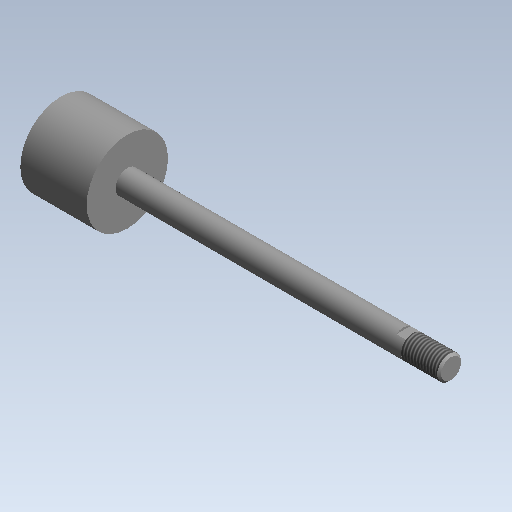
# Autodesk Inventor part: SR-092-DPY0000_rod
Saved by Autodesk Inventor 2020 (Build 240168000, 168)
## iProperties
Part Number: SR-092-DPY0000_rod
Material: Generic
Catalog Web Link: www.cadenas.de
Description: Standard Air Cylinder_rod-Original Line - Standard Air Cylinders
Vendor: BIMBA
Document SubType Name: Modeling
Designer: partserver
Manufacturer: BIMBA
Mass: 18.0803 g
Surface Area: 57.2606 cm^2
Volume: 18.0803 cm^3
Density: 1 g/cm^3
Appearance: PSOLRGB-181-181-181
Category: PARTsolutions
Company: BIMBA
PSOL_IDENT_0: {$CADENAS_DATA\23d-libs\bimba\bimba_brand\bimba_imperial\bimba_full_line\original_line_cylinders\sta
PSOL_IDENT_1: ndard_air_cylinders\rod.prj},337 {VTYP=3D},{NB=SR-092-DPY0000_rod},{LINA=SR-092-DPY0000_rod},{NN=Sta
PSOL_IDENT_2: ndard Air Cylinder_rod},{DATE=19.01.2022 10:19:37},{GEOMDATE=27.08.2019 11:00:52},{VERSION=},{LINEID=
PSOL_IDENT_3: 10},{WBVAR=STROKE,ACTING,MNT,DER,NR,BM,CO,M,EE,EEL,K,Q,Y,F,G,T,B,H,SER,SR,NT,W,E,HL,ST,STP,PRC,PB,CO
PSOL_IDENT_4: LOR1,FCD,RCD,BCD,ZHJ},{WBNUMERIC=STROKE,EEL,COLOR1,FCD,RCD,BCD,ZHJ}  {NB=SR-092-DPY0000_rod},{LINA=S
PSOL_IDENT_5: R-092-DPY0000_rod},{KT=DUMMY},{PN=SR-092-DPY000},{DASH=-},{BORE=1.06250000},{BOREPN=09},{STROKE=2.00
PSOL_IDENT_6: 0},{STROKEALG=[0.001:50/0.001]},{STROKE1=2.000},{ACTING=D},{ACTINGALG= '' , 'Single Acting' , 'R' , '
PSOL_IDENT_7: Reverse Single Acting' , 'D' , 'Double Acting' },{ACTINGPN=D},{MNT=P},{MNTALG= '' , 'Front Nose Moun
PSOL_IDENT_8: ting' , 'P' , 'Rear Pivot Mounting' , 'X' , 'Universal Pivot Mounting or Double End Mounting' , 'BF'
PSOL_IDENT_9: , 'Front Block Mounting' , 'BR' , 'Rear Block Mounting for Vertical Positioning' , 'BFT' , 'Front B
PSOL_IDENT_10: lock Trunnion Mounting' , 'BRT' , 'Rear Block Trunnion Mounting' },{TYPE=SR-},{MNTPN=P},{DER=},{DERA
PSOL_IDENT_11: LG= '' , 'N/A' },{NR=},{NRALG= '' , 'N/A' },{NRPN=},{BM=},{BMALG= '' , 'N/A' },{BMPN=},{CO=},{COALG=
PSOL_IDENT_12: '' , 'N/A' },{M=},{MALG= '', 'Without Magnet', 'M', 'With Magnet' },{EE=},{EEL=0},{EEMAX=48},{EEALG=
PSOL_IDENT_13: '', 'Without Extra Extension', 'EE', 'With Extra Extension' },{EELALG=0},{EEPN=},{EEPN1=0.000},{K=}
PSOL_IDENT_14: ,{KALG= '', 'Standard' , 'K' , 'Ports Rotated 90deg' },{KPN=},{Q=},{QALG= '' , 'Without Side Ported
PSOL_IDENT_15: Rear Head' , 'Q' , 'With Side Ported Rear Head' },{QPN=},{Y=Y},{YALG= '' , 'Without Pivot Bushing' ,
PSOL_IDENT_16: 'Y' , 'With Pivot Bushing' },{YPN=Y},{F=},{FALG= '', 'Standard', 'F', 'Molycoated Body' },{FPN=},{G=
PSOL_IDENT_17: },{GPN=},{T=},{TALG= '' , 'Standard' , 'N' , 'Low Temperature' , 'V' , 'High Temperature' },{NPN=},{
PSOL_IDENT_18: VPN=},{B=},{BALG= '', 'Without Bumper' , 'B' , 'With Bumper' },{BPN=},{H=},{HALG= '', 'N/A' },{HPN=}
PSOL_IDENT_19: ,{SER=},{SERALG= '' , 'Without Spring Extend/Return' , 'JS' , 'With Spring Return' , 'JR' , 'With Sp
PSOL_IDENT_20: ring Extend' },{SR=SR},{SRALG= 'C' , 'Carbon Steel Rod' , 'SR' , '303 Stainless Steel Rod' , '' , '3
PSOL_IDENT_21: 03 Stainless Steel Rod1' },{SRPN=SR},{SRCON=1},{NT=},{NTPN=},{W=},{WALG= '' , 'Without Wiper' , 'W'
PSOL_IDENT_22: , 'With Wiper' },{WPN=},{E=},{EALG= '' , 'Without Special Lube and Seals' , 'E' , 'With Special Lube
PSOL_IDENT_23: and Seals' },{EPN=},{HL=},{HLALG= '' , 'Wihout Low Pressure Hydraulic' , 'HL' , 'With Low Pressure
PSOL_IDENT_24: Hydraulic' },{ST=},{STALG= '' , 'Without Switch Track' , 'T' , 'With Switch Track' },{STP=},{STPALG=
PSOL_IDENT_25: '' , 'N/A' },{STPN=},{PRC=},{PRCALG= '' , 'Without Piston Rod Clevis' , 'D-166-1' , 'With Piston Ro
PSOL_IDENT_26: d Clevis' },{PRCPN=},{PB=},{PBALG= '' , 'Without Pivot Bracket' , 'D-167' , 'With Pivot Bracket' },{
PSOL_IDENT_27: PBPN=},{TLEN=3.3135},{TEXT=0.233333},{SPACE=0.133333},{FRAC=8.8400},{RGCON=},{RGDACCON=R},{RHCON=P},
PSOL_IDENT_28: {RHCONON=1},{RHACCON=},{FNUTCON=0},{RNUTCON=0},{FNUTPN=},{RNUTPN=},{FNUTTRANS=0.0000},{RNUTTRANS=0.0
PSOL_IDENT_29: 000},{VHOLECON=0},{A1=1.6250},{A1N=1.0000},{A1P=1.6250},{A1B=1.8750},{A4=0.2525},{A4N=0.3750},{A4P=0
PSOL_IDENT_30: .2525},{A5=0.0300},{A1H=1.5},{A1NH=0.6250},{A1PH=1.5000},{A1BH=1.1250},{A1SH=1.1250},{A2H=0.2500},{A
PSOL_IDENT_31: 2NH=0.2500},{LENGTH=3.8400},{LENGTH1=3.8400},{LENGTH2=4.1000},{MUL=2.0000},{MUL11=2.0000},{MUL22=5.1
PSOL_IDENT_32: 200},{MUL33=3.1200},{MUL2=2.0000},{MUL211=2.0000},{MUL222=2.5600},{MUL233=1.5600},{SSS=4.0000},{RGLE
PSOL_IDENT_33: N=1.4025},{RHLEN=0.9990},{SSS1=3.0000},{A13=1.2190},{THDLEN1=0.5000},{THD1=0.3125},{TAB=UNF},{THDLEN=
PSOL_IDENT_34: 0.5000},{THD=0.3125},{OD=1.0715},{RODL=5.1210},{PL=0.8710},{RODDIA=0.3120},{HEX=0.3750},{RODTRANS=0.
PSOL_IDENT_35: 0000},{G1=0.3440},{ON=0},{G5=0.7180},{DERLEN=4.1250},{THOLE=0.1700},{WF=0.2500},{BADD=0.0000},{MADD=
PSOL_IDENT_36: 0.0000},{NVADD=0.000},{JRADD=0.00000},{COLOR=0.71,0.71,0.71,0.00},{GROOVE=1},{HOL=0},{D7=0.2520},{H1=
PSOL_IDENT_37: 0.0000},{D1=1.1130},{D1RH=1.1110},{D1P=1.1410},{D1B=1.1130},{D1N=1.1130},{D1NRH=1.1155},{D1BRH=1.141
PSOL_IDENT_38: 0},{D1PRH=1.1110},{BOZO=0},{HADD=0.000},{COLOR1=0},{DEFL=0.0000},{HEXL=0.0000},{SSADD=0.0000},{WFL=0
PSOL_IDENT_39: .1250},{MOVE=0.1250},{PRCL2=0.50000},{PRCB=0.19000},{PRCTRANS=0.19000},{FCD=0},{RCD=0},{BCD=0},{ZHJ=
PSOL_IDENT_40: 0.000}
NB: SR-092-DPY0000_rod
NN: Standard Air Cylinder_rod
NT: Standard
NBSYN: $PN.$COLOR1._rod
LINA: SR-092-DPY0000_rod
CATALOG: Bimba Products
PN: SR-092-DPY000
BORE: 1.0625
BOREPN: 09
STROKE: 2
ACTING: Double Acting
MNT: Rear Pivot Mounting
DER: N/A
NR: N/A
BM: N/A
CO: N/A
M: Without Magnet
EE: Without Extra Extension
EEL: 0
K: Standard
Q: Without Side Ported Rear Head
Y: With Pivot Bushing
F: Standard
G: Without Magnalube Lubrication
T: Standard
B: Without Bumper
H: N/A
SER: Without Spring Extend/Return
SR: 303 Stainless Steel Rod
W: Without Wiper
E: Without Special Lube and Seals
HL: Wihout Low Pressure Hydraulic
ST: Without Switch Track
STP: N/A
PRC: Without Piston Rod Clevis
PB: Without Pivot Bracket
A1N: 1
A1P: 1.625
A1B: 1.875
A4N: 0.375
A4P: 0.2525
A5: 0.03
A1NH: 0.625
A1PH: 1.5
A1BH: 1.125
A1SH: 1.125
A2NH: 0.25
A13: 1.219
THDLEN1: 0.5
THD1: 0.3125
TAB: UNF
OD: 1.0715
RODDIA: 0.312
HEX: 0.375
G1: 0.344
G5: 0.718
THOLE: 0.17
WF: 0.25
GROOVE: 1
D7: 0.252
D1P: 1.141
D1B: 1.113
D1N: 1.113
D1NRH: 1.1155
D1BRH: 1.141
D1PRH: 1.111
COLOR1: 0
FCD: 0
RCD: 0
BCD: 0
ZHJ: 0
SUPPLIER: BIMBA
ARTICLENO: SR-092-DPY0000_rod
BOMINFO: SR-092-DPY0000_rod
CREATOR: CADENAS GmbH
Title: SR-092-DPY0000_rod
Author: Cadenas PARTsolutions
Comments: Original Line - Standard Air Cylinders
Autodesk Inventor part; units mm, degrees
sketch "Sketch_1" plane through (0, 0, 0) normal (0, 0, 1) x (1, 0, 0)
  line L0 (114.1984, 0) -> (-3.175, 0)
  line L1 (-3.175, 0) -> (-3.175, 3.9624)
  line L2 (-3.175, 3.9624) -> (92.075, 3.9624)
  line L3 (92.075, 3.9624) -> (92.075, 13.5572)
  line L4 (92.075, 13.5572) -> (114.1984, 13.5572)
  line L5 (114.1984, 13.5572) -> (114.1984, 0)
  line L6 (114.1984, 0) -> (-3.175, 0)
  constraints: 14 end point
revolve "Revolution1" add sketch "Sketch_1" angle 360 about axis through (114.1984, 0, 0) along (1, 0, 0)
sketch "Sketch_3" plane through (0, 0, 0) normal (0, 0, 1) x (1, 0, 0)
  line L0 (-3.175, 0) -> (-15.875, 0)
  line L1 (-15.875, 0) -> (-15.875, 3.3388)
  line L2 (-15.875, 3.3388) -> (-15.2451, 3.9688)
  line L3 (-15.2451, 3.9688) -> (-3.175, 3.9688)
  line L4 (-3.175, 3.9688) -> (-3.175, 0)
  line L5 (-3.175, 0) -> (-15.875, 0)
  constraints: 12 end point
revolve "Revolution2" add sketch "Sketch_3" angle 360 about axis through (-3.175, 0, 0) along (1, 0, 0)
thread "Thread1" size "5/16-24 UNF" class "2A" standard "ANSI Unified Screw Threads" full length
sketch "Sketch_10" plane through (-3.175, 0, 0) normal (1, 0, 0) x (0, 0, -1)
  line L0 (-7.9248, -7.9248) -> (7.9248, -7.9248)
  line L1 (7.9248, -7.9248) -> (7.9248, 7.9248)
  line L2 (7.9248, 7.9248) -> (-7.9248, 7.9248)
  line L3 (-7.9248, 7.9248) -> (-7.9248, -7.9248)
  line L4 (-3.175, -3.9624) -> (3.175, -3.9624)
  line L5 (3.175, -3.9624) -> (3.175, 3.9624)
  line L6 (3.175, 3.9624) -> (-3.175, 3.9624)
  line L7 (-3.175, 3.9624) -> (-3.175, -3.9624)
  constraints: 16 end point
extrude "Extrusion1" cut sketch "Sketch_10" along normal blind 3.175
ref_plane "dia1_XY" through (-3.175, 3.9624, 0) normal (1, 0, 0) x (0, 0, -1)
ref_plane "dia1_YZ" through (-3.175, 3.9624, 0) normal (0, 0, -1) x (0, 1, 0)
ref_plane "dia1_ZX" through (-3.175, 3.9624, 0) normal (0, 1, 0) x (1, 0, 0)
ref_plane "dia12_XY" through (0, 0, 14.1351) normal (1, 0, 0) x (0, 0, -1)
ref_plane "dia12_YZ" through (0, 0, 14.1351) normal (0, 0, -1) x (0, 1, 0)
ref_plane "dia12_ZX" through (0, 0, 14.1351) normal (0, 1, 0) x (1, 0, 0)
ref_plane "dia2_XY" through (-3.175, -3.9624, 0) normal (1, 0, 0) x (0, 0, -1)
ref_plane "dia2_YZ" through (-3.175, -3.9624, 0) normal (0, 0, -1) x (0, 1, 0)
ref_plane "dia2_ZX" through (-3.175, -3.9624, 0) normal (0, 1, 0) x (1, 0, 0)
ref_plane "dia22_XY" through (0, 0, -14.1351) normal (1, 0, 0) x (0, 0, -1)
ref_plane "dia22_YZ" through (0, 0, -14.1351) normal (0, 0, -1) x (0, 1, 0)
ref_plane "dia22_ZX" through (0, 0, -14.1351) normal (0, 1, 0) x (1, 0, 0)
ref_plane "rl1_XY" through (-15.875, 0, 0) normal (1, 0, 0) x (0, 0, -1)
ref_plane "rl1_YZ" through (-15.875, 0, 0) normal (0, 0, -1) x (0, 1, 0)
ref_plane "rl1_ZX" through (-15.875, 0, 0) normal (0, 1, 0) x (1, 0, 0)
ref_plane "rl2_XY" through (-3.175, 0, 0) normal (1, 0, 0) x (0, 0, -1)
ref_plane "rl2_YZ" through (-3.175, 0, 0) normal (0, 0, -1) x (0, 1, 0)
ref_plane "rl2_ZX" through (-3.175, 0, 0) normal (0, 1, 0) x (1, 0, 0)
ref_plane "rod_cp_XY" through (0, 0, 0) normal (1, 0, 0) x (0, 0, -1)
ref_plane "rod_cp_YZ" through (0, 0, 0) normal (0, 0, -1) x (0, 1, 0)
ref_plane "rod_cp_ZX" through (0, 0, 0) normal (0, 1, 0) x (1, 0, 0)
ref_plane "thd1_XY" through (-15.875, 3.9688, 0) normal (1, 0, 0) x (0, 0, -1)
ref_plane "thd1_YZ" through (-15.875, 3.9688, 0) normal (0, 0, -1) x (0, 1, 0)
ref_plane "thd1_ZX" through (-15.875, 3.9688, 0) normal (0, 1, 0) x (1, 0, 0)
ref_plane "thd2_XY" through (-15.875, -3.9688, 0) normal (1, 0, 0) x (0, 0, -1)
ref_plane "thd2_YZ" through (-15.875, -3.9688, 0) normal (0, 0, -1) x (0, 1, 0)
ref_plane "thd2_ZX" through (-15.875, -3.9688, 0) normal (0, 1, 0) x (1, 0, 0)
ref_plane "to_rod_clevis_XY" through (-20.701, 0, 0) normal (1, 0, 0) x (0, 0, -1)
ref_plane "to_rod_clevis_YZ" through (-20.701, 0, 0) normal (0, 0, -1) x (0, 1, 0)
ref_plane "to_rod_clevis_ZX" through (-20.701, 0, 0) normal (0, 1, 0) x (1, 0, 0)
ref_plane "wf1_XY" through (-3.175, 0, 0) normal (1, 0, 0) x (0, 0, -1)
ref_plane "wf1_YZ" through (-3.175, 0, 0) normal (0, 0, -1) x (0, 1, 0)
ref_plane "wf1_ZX" through (-3.175, 0, 0) normal (0, 1, 0) x (1, 0, 0)
ref_plane "wf2_XY" through (0, 0, 0) normal (1, 0, 0) x (0, 0, -1)
ref_plane "wf2_YZ" through (0, 0, 0) normal (0, 0, -1) x (0, 1, 0)
ref_plane "wf2_ZX" through (0, 0, 0) normal (0, 1, 0) x (1, 0, 0)
ref_plane "wfw1_XY" through (-3.175, 0, -3.175) normal (0, 1, 0) x (1, 0, 0)
ref_plane "wfw1_YZ" through (-3.175, 0, -3.175) normal (1, 0, 0) x (0, 0, -1)
ref_plane "wfw1_ZX" through (-3.175, 0, -3.175) normal (0, 0, -1) x (0, 1, 0)
ref_plane "wfw2_XY" through (-3.175, 0, 3.175) normal (0, 1, 0) x (1, 0, 0)
ref_plane "wfw2_YZ" through (-3.175, 0, 3.175) normal (1, 0, 0) x (0, 0, -1)
ref_plane "wfw2_ZX" through (-3.175, 0, 3.175) normal (0, 0, -1) x (0, 1, 0)
body "Solid1"
